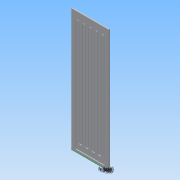
# Autodesk Inventor part: Sign ply back, v3 separate parts
Saved by Autodesk Inventor 2013 (Build 170138000, 138)
## iProperties
Created: 2018-07-07
Part Number: Sign ply back, v3 separate parts
Material: Generic
Document SubType Name: Modeling
Designer: Jeff Vyduna
Density: 1 g/cm^3
Author: Jeff Vyduna
Autodesk Inventor part; units mm, degrees
ref_plane "YZ Plane" through (0, 0, 0) normal (1, 0, 0) x (0, 1, 0)
ref_plane "XZ Plane" through (0, 0, 0) normal (0, 1, 0) x (-1, 0, 0)
ref_plane "XY Plane" through (0, 0, 0) normal (0, 0, 1) x (1, 0, 0)
sketch "TwoLineColumn" plane through (0, 0, 0) normal (0, 0, 1) x (1, 0, 0)
  line L0 (50.8, -753.9609) -> (50.8, 922.4391) construction
  line L1 (101.6, -753.9609) -> (101.6, 922.4391) construction
  arc A0 (101.6, 922.4391) -> (50.8, 922.4391) centre (76.2, 922.4391) ccw construction
  arc A1 (101.6, -753.9609) -> (152.4, -753.9609) centre (127, -753.9609) ccw construction
  line L2 (56.896, -753.9609) -> (56.896, 922.4391)
  arc A2 (95.504, 922.4391) -> (56.896, 922.4391) centre (76.2, 922.4391) ccw
  line L3 (95.504, 922.4391) -> (95.504, -753.9609)
  arc A3 (95.504, -753.9609) -> (158.496, -753.9609) centre (127, -753.9609) ccw
  line L4 (44.704, -753.9609) -> (44.704, 922.4391)
  arc A4 (107.696, 922.4391) -> (44.704, 922.4391) centre (76.2, 922.4391) ccw
  line L5 (107.696, 922.4391) -> (107.696, -753.9609)
  arc A5 (107.696, -753.9609) -> (146.304, -753.9609) centre (127, -753.9609) ccw
  line L6 (50.8, -753.9609) -> (152.4, -753.9609) construction
  dimension "d4" = 1676.4
  dimension "lineSpacing" = 50.8
  dimension "d6" = 25.4
  dimension "d9" = 6.096
  dimension "d10" = 6.096
  measures "d4" distance of L0.start L0.end
  measures "lineSpacing" distance between parallel lines of L1 L0
  measures "d6" radius of A1
  measures "d9" distance between parallel lines of L1 L3
  measures "d10" distance between parallel lines of L5 L1
sketch "TwoLineColumnEnd" plane through (0, 0, 0) normal (0, 0, 1) x (1, 0, 0)
  line L0 (103.0524, -945.1843) -> (103.0524, 731.2157)
  arc A0 (166.0444, 731.2157) -> (103.0524, 731.2157) centre (134.5484, 731.2157) ccw
  line L1 (166.0444, 731.2157) -> (166.0444, -945.1843)
  line L2 (109.1484, -945.1843) -> (109.1484, 731.2157) construction
  line L3 (159.9484, -945.1843) -> (159.9484, 731.2157) construction
  arc A1 (159.9484, 731.2157) -> (109.1484, 731.2157) centre (134.5484, 731.2157) ccw construction
  line L4 (115.2444, -945.1843) -> (115.2444, 731.2157)
  arc A2 (153.8524, 731.2157) -> (115.2444, 731.2157) centre (134.5484, 731.2157) ccw
  line L5 (153.8524, 731.2157) -> (153.8524, -945.1843)
  line L6 (109.1484, -945.1843) -> (159.9484, -945.1843) construction
  dimension "d22" = 1676.4
  dimension "d23" = 50.8
  dimension "d25" = 6.096
  dimension "d26" = 6.096
  dimension "d29" = 50.8
  measures "d22" distance of L2.start L2.end
  measures "d23" distance between parallel lines of L3 L2
  measures "d25" distance between parallel lines of L3 L5
  measures "d26" distance between parallel lines of L1 L3
  measures "d29" distance of L2.start L6.end
sketch "15mm Neon profile" plane through (0, 0, 0) normal (0, 0, 1) x (1, 0, 0)
  circle A0 centre (522.6685, 24.7098) radius 6.985 construction
  line L0 (516.6995, 21.082) -> (528.6375, 21.082) construction
  line L1 (528.6375, 21.082) -> (528.6375, 6.35) construction
  line L2 (528.6375, 6.35) -> (516.6995, 6.35) construction
  line L3 (516.6995, 6.35) -> (516.6995, 21.082) construction
  point P0 (522.6685, 16.011)
  dimension "d73" = 13.97
  dimension "d74" = 11.938
  dimension "d76" = 14.732
  measures "d73" diameter of A0
  measures "d74" distance of L0.start L0.end
  measures "d76" distance of L0.end L1.end
sketch "Sketch1" plane through (0, 0, 0) normal (0, 0, 1) x (1, 0, 0)
  line L0 (0, 0) -> (604.8375, 0)
  line L1 (604.8375, 0) -> (604.8375, 1981.2)
  line L2 (604.8375, 1981.2) -> (0, 1981.2)
  line L3 (0, 1981.2) -> (0, 0)
  dimension "d1" = 604.8375
  dimension "d2" = 1981.2
  constraints: 8 end point, 2 parallel, 1 coincident, 1 horizontal, 1 perpendicular
  measures "d1" distance of L2.end L1.end
  measures "d2" distance of L1.end L0.end
extrude "Extrusion1" add sketch "Sketch1" along normal blind 19.05
sketch "LEDPocket" plane through (0, 0, 19.05) normal (0, 0, 1) x (1, 0, 0)
  line L0 (0, 0) -> (604.8375, 0) projected
  line L1 (604.8375, 0) -> (604.8375, 1981.2) projected
  line L2 (604.8375, 1981.2) -> (0, 1981.2) projected
  line L3 (38.1, 1981.2) -> (38.1, 0) construction
  line L4 (566.7375, 1981.2) -> (566.7375, 0) construction
  line L5 (67.564, 166.116) -> (67.564, 42.8625)
  line L6 (72.3265, 38.1) -> (532.1935, 38.1)
  line L7 (536.956, 42.8625) -> (536.956, 166.116)
  line L8 (79.756, 166.116) -> (79.756, 147.32)
  line L9 (105.156, 121.92) -> (499.364, 121.92)
  line L10 (524.764, 147.32) -> (524.764, 166.116)
  arc A0 (79.756, 147.32) -> (105.156, 121.92) centre (105.156, 147.32) ccw
  arc A1 (499.364, 121.92) -> (524.764, 147.32) centre (499.364, 147.32) ccw
  arc A2 (67.564, 42.8625) -> (72.3265, 38.1) centre (72.3265, 42.8625) ccw
  arc A3 (532.1935, 38.1) -> (536.956, 42.8625) centre (532.1935, 42.8625) ccw
  line L11 (473.964, 166.116) -> (473.964, 1842.516)
  arc A4 (536.956, 1842.516) -> (473.964, 1842.516) centre (505.46, 1842.516) ccw
  line L12 (536.956, 1842.516) -> (536.956, 166.116)
  line L13 (480.06, 166.116) -> (480.06, 1842.516) construction
  line L14 (530.86, 166.116) -> (530.86, 1842.516) construction
  arc A5 (530.86, 1842.516) -> (480.06, 1842.516) centre (505.46, 1842.516) ccw construction
  line L15 (486.156, 166.116) -> (486.156, 1842.516)
  arc A6 (524.764, 1842.516) -> (486.156, 1842.516) centre (505.46, 1842.516) ccw
  line L16 (524.764, 1842.516) -> (524.764, 166.116)
  line L17 (480.06, 166.116) -> (530.86, 166.116) construction
  line L18 (67.564, 166.116) -> (67.564, 1842.516)
  arc A7 (130.556, 1842.516) -> (67.564, 1842.516) centre (99.06, 1842.516) ccw
  line L19 (130.556, 1842.516) -> (130.556, 166.116)
  arc A8 (130.556, 166.116) -> (169.164, 166.116) centre (149.86, 166.116) ccw
  line L20 (73.66, 166.116) -> (73.66, 1842.516) construction
  line L21 (124.46, 166.116) -> (124.46, 1842.516) construction
  arc A9 (124.46, 1842.516) -> (73.66, 1842.516) centre (99.06, 1842.516) ccw construction
  arc A10 (124.46, 166.116) -> (175.26, 166.116) centre (149.86, 166.116) ccw construction
  line L22 (79.756, 166.116) -> (79.756, 1842.516)
  arc A11 (118.364, 1842.516) -> (79.756, 1842.516) centre (99.06, 1842.516) ccw
  line L23 (118.364, 1842.516) -> (118.364, 166.116)
  arc A12 (118.364, 166.116) -> (181.356, 166.116) centre (149.86, 166.116) ccw
  line L24 (73.66, 166.116) -> (175.26, 166.116) construction
  line L25 (169.164, 166.116) -> (169.164, 1842.516)
  arc A13 (232.156, 1842.516) -> (169.164, 1842.516) centre (200.66, 1842.516) ccw
  line L26 (232.156, 1842.516) -> (232.156, 166.116)
  arc A14 (232.156, 166.116) -> (270.764, 166.116) centre (251.46, 166.116) ccw
  line L27 (175.26, 166.116) -> (175.26, 1842.516) construction
  line L28 (226.06, 166.116) -> (226.06, 1842.516) construction
  arc A15 (226.06, 1842.516) -> (175.26, 1842.516) centre (200.66, 1842.516) ccw construction
  arc A16 (226.06, 166.116) -> (276.86, 166.116) centre (251.46, 166.116) ccw construction
  line L29 (181.356, 166.116) -> (181.356, 1842.516)
  arc A17 (219.964, 1842.516) -> (181.356, 1842.516) centre (200.66, 1842.516) ccw
  line L30 (219.964, 1842.516) -> (219.964, 166.116)
  arc A18 (219.964, 166.116) -> (282.956, 166.116) centre (251.46, 166.116) ccw
  line L31 (270.764, 166.116) -> (270.764, 1842.516)
  arc A19 (333.756, 1842.516) -> (270.764, 1842.516) centre (302.26, 1842.516) ccw
  line L32 (333.756, 1842.516) -> (333.756, 166.116)
  arc A20 (333.756, 166.116) -> (372.364, 166.116) centre (353.06, 166.116) ccw
  line L33 (276.86, 166.116) -> (276.86, 1842.516) construction
  line L34 (327.66, 166.116) -> (327.66, 1842.516) construction
  arc A21 (327.66, 1842.516) -> (276.86, 1842.516) centre (302.26, 1842.516) ccw construction
  arc A22 (327.66, 166.116) -> (378.46, 166.116) centre (353.06, 166.116) ccw construction
  line L35 (282.956, 166.116) -> (282.956, 1842.516)
  arc A23 (321.564, 1842.516) -> (282.956, 1842.516) centre (302.26, 1842.516) ccw
  line L36 (321.564, 1842.516) -> (321.564, 166.116)
  arc A24 (321.564, 166.116) -> (384.556, 166.116) centre (353.06, 166.116) ccw
  line L37 (372.364, 166.116) -> (372.364, 1842.516)
  arc A25 (435.356, 1842.516) -> (372.364, 1842.516) centre (403.86, 1842.516) ccw
  line L38 (435.356, 1842.516) -> (435.356, 166.116)
  arc A26 (435.356, 166.116) -> (473.964, 166.116) centre (454.66, 166.116) ccw
  line L39 (378.46, 166.116) -> (378.46, 1842.516) construction
  line L40 (429.26, 166.116) -> (429.26, 1842.516) construction
  arc A27 (429.26, 1842.516) -> (378.46, 1842.516) centre (403.86, 1842.516) ccw construction
  arc A28 (429.26, 166.116) -> (480.06, 166.116) centre (454.66, 166.116) ccw construction
  line L41 (384.556, 166.116) -> (384.556, 1842.516)
  arc A29 (423.164, 1842.516) -> (384.556, 1842.516) centre (403.86, 1842.516) ccw
  line L42 (423.164, 1842.516) -> (423.164, 166.116)
  arc A30 (423.164, 166.116) -> (486.156, 166.116) centre (454.66, 166.116) ccw
  point P0 (67.564, 38.1)
  dimension "d7" = 73.66
  dimension "d18" = 38.1
  dimension "d19" = 1981.2
  dimension "d20" = 1981.2
  dimension "d21" = 566.7375
  dimension "d31" = 38.1
  dimension "d32" = 83.82
  dimension "d33" = 44.196
  dimension "d34" = 25.4
  dimension "d35" = 4.7625
  dimension "d37" = 138.684
  dimension "d38" = 166.116
  dimension "d41" = 1676.4
  dimension "d42" = 50.8
  dimension "d43" = 6.096
  dimension "d44" = 6.096
  dimension "d45" = 50.8
  dimension "d49" = 1676.4
  dimension "d50" = 50.8
  dimension "d51" = 25.4
  dimension "d52" = 6.096
  dimension "d53" = 6.096
  constraints: 80 end point, 62 point on circle, 31 centre point, 31 tangent, 24 vertical, 22 parallel, 16 horizontal alignment, 8 equal radius, 5 perpendicular, 2 point on line, 1 coincident, 10 other
  measures "d7" distance from line of L20 point (0, 0)
  measures "d18" distance from line of point (0, 0) L3
  measures "d19" distance of L3.start L3.end
  measures "d20" distance of L4.start L4.end
  measures "d21" distance from line of L0.start L4
  measures "d31" vertical distance of L0.start point (67.564, 38.1)
  measures "d32" distance between parallel lines of L6 L9
  measures "d33" distance from line of L20.start L9
  measures "d34" radius of A0
  measures "d35" radius of A2
  measures "d37" distance from line of A7.centre L2
  measures "d38" distance from line of L20.start L0
  measures "d41" distance of L13.start L13.end
  measures "d42" distance between parallel lines of L14 L13
  measures "d43" distance between parallel lines of L14 L16
  measures "d44" distance between parallel lines of L12 L14
  measures "d45" distance of L13.start L17.end
  measures "d49" distance of L20.start L20.end
  measures "d50" distance between parallel lines of L21 L20
  measures "d51" radius of A10
  measures "d52" distance between parallel lines of L21 L23
  measures "d53" distance between parallel lines of L19 L21
extrude "Extrusion3" cut sketch "LEDPocket" against normal blind 12.7
sketch "Sketch5" plane through (0, 0, 0) normal (0, -1, 0) x (1, 0, 0)
  line L0 (0, 0) -> (604.8375, 0) projected
  line L1 (604.8375, 0) -> (604.8375, 19.05) projected
  line L2 (566.7375, 38.1) -> (566.7375, 19.05) projected
  line L3 (0, 19.05) -> (604.8375, 19.05) projected
  line L4 (0, 0) -> (0, 19.05) projected
  line L5 (566.7375, 32.05) -> (522.6685, 32.05) construction
  line L6 (598.4875, 38.1) -> (586.2955, 38.1) construction
  line L7 (586.2955, 38.1) -> (586.2955, 25.4) construction
  line L8 (586.2955, 25.4) -> (598.4875, 25.4) construction
  line L9 (598.4875, 25.4) -> (598.4875, 38.1) construction
  line L10 (566.7375, 39.6382) -> (576.2625, 39.6382)
  line L11 (576.2625, 39.6382) -> (576.2625, 34.4312)
  line L12 (576.2625, 34.4312) -> (566.7375, 34.4312)
  line L13 (566.7375, 34.4312) -> (566.7375, 39.6382)
  circle A0 centre (522.6685, 24.7098) radius 6.985 construction
  line L14 (516.6995, 21.082) -> (528.6375, 21.082) construction
  line L15 (528.6375, 21.082) -> (528.6375, 6.35) construction
  line L16 (528.6375, 6.35) -> (516.6995, 6.35) construction
  line L17 (516.6995, 6.35) -> (516.6995, 21.082) construction
  circle A1 centre (592.3915, 43.7598) radius 6.985 construction
  line L18 (586.4225, 40.132) -> (598.3605, 40.132) construction
  line L19 (598.3605, 40.132) -> (598.3605, 25.4) construction
  line L20 (598.3605, 25.4) -> (586.4225, 25.4) construction
  line L21 (586.4225, 25.4) -> (586.4225, 40.132) construction
  point P0 (592.3915, 25.4)
  point P1 (592.3915, 25.4)
  dimension "d75" = 12.7
  dimension "d79" = 38.1
  dimension "d80" = 12.192
  dimension "d81" = 12.7
  dimension "d83" = 13
  dimension "d84" = 9.525
  dimension "d85" = 5.207
  dimension "d86" = 15.3812
  dimension "d87" = 28.0813
  dimension "d88" = 6.35
  constraints: 18 end point, 4 horizontal, 4 parallel, 2 perpendicular, 2 point on line, 1 coincident, 1 midpoint, 2 other
  measures "d80" distance of L8.end L7.end
  measures "d81" distance of L7.end L6.end
  measures "d83" distance of L2.end L5.start
  measures "d84" distance of L11.end L12.end
  measures "d85" distance of L10.end L11.end
  measures "d86" distance of L12.end L2.end
  measures "d88" horizontal distance of L1.end L8.end
equation "\"d18\" = borderW"
equation "\"d31\" = borderW"
equation "\"d4\" = litH"
equation "\"d6\" = 0.5 * lineSpacing"
equation "\"d9\" = 0.5 * pathW"
equation "\"d10\" = 0.5 * pathW"
equation "\"d22\" = litH"
equation "\"d25\" = 0.5 * pathW"
equation "\"d26\" = 0.5 * pathW"
equation "\"d29\" = lineSpacing"
equation "\"d1\" = signW"
equation "\"d2\" = signH"
equation "\"d19\" = signH"
equation "\"d20\" = signH"
equation "\"d21\" = signW - borderW"
equation "\"d32\" = ePocketH"
equation "\"d33\" = litHClearanceH"
equation "\"d34\" = minBendR"
equation "\"d35\" = 0.5 * pathEndMillD"
equation "\"d41\" = d46"
equation "\"d43\" = 0.5 * d48"
equation "\"d44\" = 0.5 * d48"
equation "\"d45\" = d47"
equation "\"d49\" = d54"
equation "\"d51\" = 0.5 * d50"
equation "\"d52\" = 0.5 * d55"
equation "\"d53\" = 0.5 * d55"
equation "\"d79\" = borderPadding + 0.5 * lineSpacing"
equation "\"litH\" = 1676.4"
equation "\"borderW\" = 38.1"
equation "\"pathEndMillD\" = 9.525"
equation "\"signW\" = -0.5 * pathEndMillD + 0.5 * ply4x8w"
equation "\"pathW\" = 12.192"
equation "\"ply4x8w\" = 1219.2"
equation "\"signH\" = 1981.2"
equation "\"borderPadding\" = 12.7"
equation "\"ePocketH\" = 83.82"
equation "\"minBendR\" = 25.4"
equation "\"d46\" = 1676.4"
equation "\"d48\" = 12.192"
equation "\"d54\" = 1676.4"
equation "\"d55\" = 12.192"
equation "\"litHClearanceH\" = 44.196"
equation "\"d47\" = 50.8"
body "Solid1"
